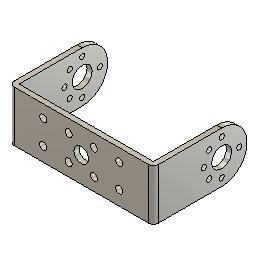
RDS3235 v8 (Autodesk Fusion 360 archive; units mm, degrees)
design "Support_large"
Autodesk Fusion 360 part; units mm, degrees
sketch "Sketch1" plane through (0, 0, 0) normal (0, 1, 0) x (1, 0, 0)
  line L0 (28.5, -18.45) -> (-28.5, -18.45)
  line L1 (-28.5, -18.45) -> (-28.5, 18.45)
  line L2 (-28.5, 18.45) -> (28.5, 18.45)
  line L3 (28.5, 18.45) -> (28.5, -18.45)
  line L4 (28.5, -18.45) -> (-28.5, 18.45) construction
  line L5 (-28.5, -18.45) -> (28.5, 18.45) construction
  line L6 (26.5, 18.45) -> (26.5, -16.45)
  line L7 (26.5, -16.45) -> (-26.5, -16.45)
  line L8 (-26.5, -16.45) -> (-26.5, 18.45)
  dimension "d1" = 57
  dimension "d2" = 36.9
  dimension "d3" = 2
  constraint perpendicular L0 L1
  constraint parallel L0 L2
  constraint parallel L1 L3
  constraint horizontal L0
  constraint coincident L4 origin
  constraint coincident L5 origin
  measures "d1" distance of L1.end L2.end
  measures "d2" distance of L0.end L1.end
extrude "Extrude1" add sketch "Sketch1" along normal blind 20 contours L0 L1 L2 L3 L6 L7 L8
sketch "Sketch2" plane through (-28.5, 0, 0) normal (-1, 0, 0) x (0, 0, 1)
  line L0 (-18.45, 0) -> (18.45, 0)
  line L1 (18.45, 0) -> (18.45, 20)
  line L2 (18.45, 20) -> (-18.45, 20)
  line L3 (-18.45, 20) -> (-18.45, 0)
  line L4 (-18.45, 10) -> (18.45, 10) construction
  circle A0 centre (-8.45, 10) radius 3.9
  circle A1 centre (-8.45, 10) radius 10
  circle A2 centre (-8.45, 10) radius 7 construction
  circle A3 centre (-15.45, 10) radius 1
  circle A4 centre (-13.3997, 5.0503) radius 1
  circle A5 centre (-8.45, 3) radius 1
  circle A6 centre (-3.5003, 5.0503) radius 1
  circle A7 centre (-1.45, 10) radius 1
  circle A8 centre (-3.5003, 14.9497) radius 1
  circle A9 centre (-8.45, 17) radius 1
  circle A10 centre (-13.3997, 14.9497) radius 1
  dimension "d6" = 7.8
  dimension "d7" = 10
  dimension "d8" = 20
  dimension "d9" = 14
  dimension "d10" = 2
  dimension "d12" = 360
  constraint midpoint L3 L4.start
  constraint midpoint L1 L4.end
  constraint coincident L4 A0.centre
  constraint concentric A0 A1
  constraint concentric A0 A2
  constraint coincident A2 A3.centre
  constraint coincident L4 A3.centre
  measures "d6" diameter of A0
  measures "d7" distance of L4.start A0.centre
  measures "d8" diameter of A1
  measures "d9" diameter of A2
  measures "d10" diameter of A3
extrude "Extrude2" cut sketch "Sketch2" against normal blind 57 contours L0 L3 A1 | L2 L3 A1 | A0 | A3 | A5 | A6 | A7 | A8 | A9
sketch "Sketch3" plane through (0, 0, 18.45) normal (0, 0, 1) x (1, 0, 0)
  line L0 (-28.5, 0) -> (28.5, 0)
  line L1 (28.5, 0) -> (28.5, 20)
  line L2 (28.5, 20) -> (-28.5, 20)
  line L3 (-28.5, 20) -> (-28.5, 0)
  line L4 (0, 0) -> (0, 20) construction
  circle A0 centre (0, 10) radius 2.9
  line L5 (5, 5) -> (-5, 5) construction
  line L6 (-5, 5) -> (-5, 15) construction
  line L7 (-5, 15) -> (5, 15) construction
  line L8 (5, 15) -> (5, 5) construction
  line L9 (5, 5) -> (-5, 15) construction
  line L10 (-5, 5) -> (5, 15) construction
  circle A1 centre (-5, 5) radius 1.4
  circle A2 centre (5, 5) radius 1.4
  circle A3 centre (5, 15) radius 1.4
  circle A4 centre (-5, 15) radius 1.4
  line L11 (-5, 15) -> (-15, 15) construction
  line L12 (-15, 15) -> (-15, 5.6132) construction
  line L13 (-15, 5.6132) -> (-5, 5.6132) construction
  line L14 (-5, 5.6132) -> (-5, 15) construction
  circle A5 centre (-15, 5.6132) radius 1.4
  circle A6 centre (-15, 15) radius 1.4
  circle A7 centre (15, 15) radius 1.4
  circle A8 centre (15, 5.6132) radius 1.4
  line L15 (15, 5.6132) -> (5, 5.6132) construction
  line L16 (5, 15) -> (15, 15) construction
  line L17 (15, 15) -> (15, 5.6132) construction
  point P0 (0, 10)
  dimension "d15" = 5.8
  dimension "d16" = 10
  dimension "d17" = 10
  dimension "d18" = 2.8
  dimension "d20" = 360
  dimension "d21" = 10
  dimension "d22" = 2.8
  dimension "d23" = 2.8
  constraint coincident L4.start origin
  constraint midpoint L2 L4.end
  constraint midpoint L4 P0
  constraint perpendicular L5 L6
  constraint parallel L5 L7
  constraint parallel L6 L8
  constraint horizontal L5
  constraint coincident L9 P0
  constraint coincident L10 P0
  constraint coincident P0 A0.centre
  constraint coincident L5.end L6.start
  constraint horizontal L11
  constraint vertical L12
  constraint horizontal L13
  constraint vertical L14
  constraint coincident L6.end L7.start
  constraint coincident L12.end L13.start
  constraint coincident L11.end L12.start
  constraint symmetric L4 L6.end L7.end
  constraint symmetric L4 L11.end A7.centre
  constraint symmetric L4 L12.end A8.centre
  constraint symmetric L4 L13.end L15.end
  constraint symmetric L4 A5 A8
  constraint symmetric L4 A6 A7
  measures "d15" diameter of A0
  measures "d16" distance of L5.end L6.end
  measures "d17" distance of L6.end L7.end
  measures "d18" diameter of A1
  measures "d21" distance of L6.end L11.end
  measures "d22" diameter of A5
  measures "d23" diameter of A6
extrude "Extrude3" cut sketch "Sketch3" against normal blind 2 contours A0 | A1 | A2 | A3 | A4 | A5 | A6 | A7 | A8
fillet "Fillet1" radius 2 2 edges at (-28.5, 10, 18.45) (28.5, 10, 18.45)
equation "d1 = 55.8 mm + 0.9 mm + 0.3 mm"

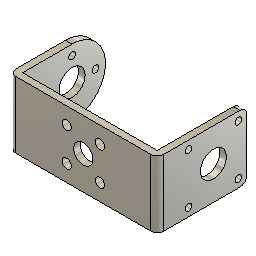
design "Support_small"
Autodesk Fusion 360 part; units mm, degrees
sketch "Sketch1" plane through (0, 0, 0) normal (0, 1, 0) x (1, 0, 0)
  line L0 (22.25, -13.45) -> (-22.25, -13.45)
  line L1 (-22.25, -13.45) -> (-22.25, 13.45)
  line L2 (-22.25, 13.45) -> (22.25, 13.45)
  line L3 (22.25, 13.45) -> (22.25, -13.45)
  line L4 (22.25, -13.45) -> (-22.25, 13.45) construction
  line L5 (-22.25, -13.45) -> (22.25, 13.45) construction
  line L6 (20.25, 13.45) -> (20.25, -11.45)
  line L7 (20.25, -11.45) -> (-20.25, -11.45)
  line L8 (-20.25, -11.45) -> (-20.25, 13.45)
  dimension "d1" = 44.5
  dimension "d2" = 26.9
  dimension "d3" = 2
  constraint perpendicular L0 L1
  constraint parallel L0 L2
  constraint parallel L1 L3
  constraint horizontal L0
  constraint coincident L4 origin
  constraint coincident L5 origin
  measures "d1" distance of L1.end L2.end
  measures "d2" distance of L0.end L1.end
extrude "Extrude1" add sketch "Sketch1" along normal blind 20 contours L0 L1 L2 L3 L6 L7 L8
sketch "Sketch2" plane through (22.25, 0, 0) normal (1, 0, 0) x (0, 0, -1)
  line L0 (-13.45, 0) -> (13.45, 0)
  line L1 (13.45, 0) -> (13.45, 20)
  line L2 (13.45, 20) -> (-13.45, 20)
  line L3 (-13.45, 20) -> (-13.45, 0)
  line L4 (13.45, 10) -> (3.45, 10) construction
  circle A0 centre (3.45, 10) radius 3.9
  line L5 (13.45, 0) -> (10.95, 0) construction
  line L6 (10.95, 0) -> (10.95, 2.5) construction
  line L7 (10.95, 2.5) -> (13.45, 2.5) construction
  line L8 (13.45, 2.5) -> (13.45, 0) construction
  line L9 (13.45, 20) -> (10.95, 20) construction
  line L10 (10.95, 20) -> (10.95, 17.5) construction
  line L11 (10.95, 17.5) -> (13.45, 17.5) construction
  line L12 (13.45, 17.5) -> (13.45, 20) construction
  circle A1 centre (10.95, 17.5) radius 1
  circle A2 centre (10.95, 2.5) radius 1
  line L13 (13.45, 2.5) -> (-15.797, 2.5) construction
  line L14 (13.45, 17.5) -> (-15.797, 17.5) construction
  circle A3 centre (-4.05, 17.5) radius 1
  circle A4 centre (-4.05, 2.5) radius 1
  dimension "d6" = 10
  dimension "d7" = 7.8
  dimension "d8" = 2.5
  dimension "d9" = 2.5
  dimension "d10" = 2.5
  dimension "d11" = 2.5
  dimension "d12" = 2
  dimension "d13" = 2
  dimension "d14" = 2
  dimension "d15" = 2
  dimension "d16" = 15
  dimension "d17" = 15
  constraint midpoint L1 L4.start
  constraint perpendicular L1 L4
  constraint coincident L4.end A0.centre
  constraint horizontal L5
  constraint vertical L6
  constraint horizontal L7
  constraint vertical L8
  constraint coincident L0.end L1.start
  constraint horizontal L9
  constraint vertical L10
  constraint horizontal L11
  constraint vertical L12
  constraint coincident L1.end L2.start
  constraint coincident L10.end L11.start
  constraint coincident L6.end L7.start
  constraint perpendicular L6 L13
  constraint perpendicular L3 L14
  constraint coincident L14 A3.centre
  constraint coincident L13 A4.centre
  measures "d6" distance of L4.start L4.end
  measures "d7" diameter of A0
  measures "d8" distance of L0.end L5.end
  measures "d9" distance of L0.end L7.end
  measures "d10" distance of L1.end L11.end
  measures "d11" distance of L1.end L9.end
  measures "d12" diameter of A1
  measures "d13" diameter of A2
  measures "d14" diameter of A3
  measures "d15" diameter of A4
  measures "d16" distance of L10.end A3.centre
  measures "d17" distance of L6.end A4.centre
extrude "Extrude2" cut sketch "Sketch2" against normal blind 2 contours A0 | A1 | A2 | A3 | A4
sketch "Sketch3" plane through (-22.25, 0, 0) normal (-1, 0, 0) x (0, 0, 1)
  line L0 (-13.45, 0) -> (13.45, 0)
  line L1 (13.45, 0) -> (13.45, 20)
  line L2 (13.45, 20) -> (-13.45, 20)
  line L3 (-13.45, 20) -> (-13.45, 0)
  line L4 (-13.45, 10) -> (-3.45, 10) construction
  circle A0 centre (-3.45, 10) radius 3.9
  circle A1 centre (-3.45, 10) radius 7 construction
  circle A2 centre (-10.45, 10) radius 1
  circle A3 centre (-3.45, 3) radius 1
  circle A4 centre (3.55, 10) radius 1
  circle A5 centre (-3.45, 17) radius 1
  circle A6 centre (-3.45, 10) radius 10
  dimension "d20" = 10
  dimension "d21" = 7.8
  dimension "d22" = 14
  dimension "d23" = 2
  dimension "d25" = 360
  constraint midpoint L3 L4.start
  constraint perpendicular L3 L4
  constraint coincident L4.end A0.centre
  constraint coincident L4 A2.centre
  constraint coincident A1 A2.centre
  constraint concentric A0 A6
  constraint coincident L4.start A6
  measures "d20" distance of L4.start L4.end
  measures "d21" diameter of A0
  measures "d22" diameter of A1
  measures "d23" diameter of A2
extrude "Extrude3" cut sketch "Sketch3" against normal blind 2 contours L0 L3 A6 | L2 L3 A6 | A0 | A2 | A3 | A4 | A5
sketch "Sketch4" plane through (0, 0, 13.45) normal (0, 0, 1) x (1, 0, 0)
  line L0 (-22.25, 0) -> (22.25, 0)
  line L1 (22.25, 0) -> (22.25, 20)
  line L2 (22.25, 20) -> (-22.25, 20)
  line L3 (-22.25, 20) -> (-22.25, 0)
  line L4 (0, 0) -> (0, 20) construction
  circle A0 centre (0, 10) radius 2.9
  line L5 (5, 5) -> (-5, 5) construction
  line L6 (-5, 5) -> (-5, 15) construction
  line L7 (-5, 15) -> (5, 15) construction
  line L8 (5, 15) -> (5, 5) construction
  line L9 (5, 5) -> (-5, 15) construction
  line L10 (-5, 5) -> (5, 15) construction
  circle A1 centre (-5, 5) radius 1.4
  circle A2 centre (5, 5) radius 1.4
  circle A3 centre (5, 15) radius 1.4
  circle A4 centre (-5, 15) radius 1.4
  point P0 (0, 10)
  dimension "d28" = 5.8
  dimension "d29" = 10
  dimension "d30" = 10
  dimension "d31" = 2.8
  dimension "d33" = 360
  constraint coincident L4.start origin
  constraint midpoint L2 L4.end
  constraint midpoint L4 P0
  constraint perpendicular L5 L6
  constraint parallel L5 L7
  constraint parallel L6 L8
  constraint horizontal L5
  constraint coincident L9 P0
  constraint coincident L10 P0
  constraint coincident P0 A0.centre
  constraint coincident L5.end L6.start
  measures "d28" diameter of A0
  measures "d29" distance of L6.end L7.end
  measures "d30" distance of L5.end L6.end
  measures "d31" diameter of A1
extrude "Extrude4" cut sketch "Sketch4" against normal blind 2 contours A0 | A1 | A2 | A3 | A4
fillet "Fillet1" radius 2 2 edges at (21.25, 20, -13.45) (21.25, 0, -13.45)
fillet "Fillet1" radius 2 2 edges at (-22.25, 10, 13.45) (22.25, 10, 13.45)
sketch "Sketch5" plane through (22.25, 10, 0) normal (1, 0, 0) x (0, 0, -1)

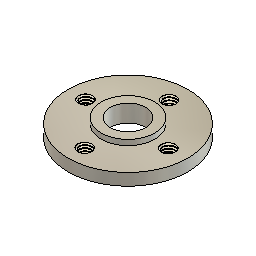
design "Wheel"
Autodesk Fusion 360 part; units mm, degrees
sketch "Sketch1" plane through (0, 0, 0) normal (0, 1, 0) x (1, 0, 0)
  circle A0 centre (0, 0) radius 10
  circle A1 centre (0, 0) radius 7 construction
  circle A2 centre (6.9997, -0.0638) radius 1.25
  circle A3 centre (0.0638, 6.9997) radius 1.25
  circle A4 centre (-6.9997, 0.0638) radius 1.25
  circle A5 centre (-0.0638, -6.9997) radius 1.25
  circle A6 centre (0, 0) radius 1.5 construction
  circle A7 centre (0, 0) radius 2.95
  circle A8 centre (0, 0) radius 4.5
  dimension "d1" = 20
  dimension "d2" = 14
  dimension "d3" = 2.5
  dimension "d5" = 360
  dimension "d6" = 3
  dimension "d7" = 5.9
  dimension "d8" = 9
  constraint coincident A0.centre A1.centre
  constraint concentric A0 A1
  constraint coincident A1 A2.centre
  constraint concentric A0 A6
  constraint concentric A0 A7
  constraint concentric A0 A8
  measures "d1" diameter of A0
  measures "d2" diameter of A1
  measures "d3" diameter of A2
  measures "d6" diameter of A6
  measures "d7" diameter of A7
  measures "d8" diameter of A8
extrude "Extrude1" add sketch "Sketch1" along normal blind 2 contours A0 | A8
extrude "Extrude2" add sketch "Sketch1" along normal blind 0.9 from surface at 2 contours A8
thread "Thread1" "ISO Metric profile 2.5 M2.5x0.45 6H" major diameter 2.58 minor diameter 2.0755 pitch 0.45 angle 60 modelled right hand crest width 0.1211 on face at (8.2482, 1.3333, 0.1261) crest through (8.0375, 0.1125, 0.0638) on face at (-5.7513, 1.3333, -0.0015) crest through (-5.962, 0.1125, -0.0638) on face at (1.3122, 1.3333, -6.9374) crest through (1.1015, 0.1125, -6.9997) on face at (1.1847, 1.3333, 7.062) crest through (0.974, 0.1125, 6.9997)
equation "d2 = 20.000 mm - 6 mm"
